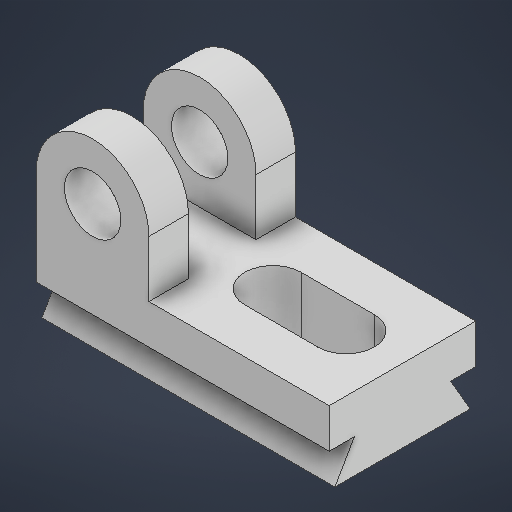
# Autodesk Inventor part: Pieza3
Saved by Autodesk Inventor 2026 (Build 300175000, 175)
## iProperties
Created: 2025-03-28
Part Number: Pieza3
Material: Genérico
Document SubType Name: Modeling
Designer: LabB305
Density: 1 g/cm^3
Appearance: Valor por defecto
Author: LabB305
Autodesk Inventor part; units mm, degrees
ref_plane "YZ Plane" through (0, 0, 0) normal (1, 0, 0) x (0, 1, 0)
ref_plane "XZ Plane" through (0, 0, 0) normal (0, 1, 0) x (-1, 0, 0)
ref_plane "XY Plane" through (0, 0, 0) normal (0, 0, 1) x (1, 0, 0)
sketch "Boceto1" plane through (0, 0, 0) normal (0, 1, 0) x (-1, 0, 0)
  point P0 (0, 0)
sketch "Boceto2" plane through (0, 0, 0) normal (1, 0, 0) x (0, 1, 0)
  line L0 (0, 0) -> (0, 12)
  line L1 (0, 0) -> (0, -12)
  line L2 (0, 0) -> (6, 0)
  line L3 (6, 0) -> (13, 0)
  line L4 (0, 12) -> (6, 8.5359)
  line L5 (0, 12) -> (6.9282, 12) construction
  line L6 (13, 0) -> (13, 13)
  line L7 (6, 8.5359) -> (6, 13)
  line L8 (6, 13) -> (13, 13)
  line L9 (13, 13) -> (33, 13)
  line L10 (33, 13) -> (33, 6)
  line L11 (33, 6) -> (13, 6)
  line L12 (0, 0) -> (0, -12)
  line L13 (0, -12) -> (6, -8.5359)
  line L14 (0, -12) -> (6.9282, -12) construction
  line L15 (13, 0) -> (13, -13)
  line L16 (6, -8.5359) -> (6, -13)
  line L17 (6, -13) -> (13, -13)
  line L18 (13, -13) -> (33, -13)
  line L19 (33, -13) -> (33, -6)
  line L20 (33, -6) -> (13, -6)
  dimension "d0" = 12
  dimension "d1" = 12
  dimension "d2" = 6
  dimension "d3" = 7
  dimension "d4" = 30
  dimension "d5" = 13
  dimension "d6" = 20
  dimension "d7" = 7
  constraints: 42 end point, 7 symmetric about line, 4 vertical, 3 horizontal, 3 perpendicular, 3 point on line, 1 equal length
  measures "d0" distance of L0.start L0.end
  measures "d1" distance of L0.start L1.end
  measures "d2" distance of L0.start L2.end
  measures "d3" distance of L2.end L3.end
  measures "d4" angle of L4 L5
  measures "d5" distance of L3.end L6.end
  measures "d6" distance of L6.end L9.end
  measures "d7" distance of L9.end L10.end
extrude "Extrusión1" add sketch "Boceto2" along normal blind 52 contours L2 L3 L15 L17 L16 L13 L1 | L0 L4 L7 L8 L6 L3 L2
sketch "Boceto3" plane through (0, 13, 13) normal (0, 1, 0) x (1, 0, 0)
  line L0 (52, 1) -> (52, 25) projected
  line L1 (52, 13) -> (42, 13)
  line L2 (42, 13) -> (29, 13)
  circle A0 centre (29, 13) radius 5
  circle A1 centre (42, 13) radius 5
  line L3 (29, 8) -> (42, 8)
  line L4 (29, 18) -> (42, 18)
  point P0 (0, 13)
  dimension "d10" = 10
  dimension "d11" = 13
  dimension "d12" = 10
  dimension "d13" = 10
  constraints: 8 end point, 4 point on circle, 2 centre point, 2 coincident, 2 tangent, 1 horizontal, 1 midpoint, 1 parallel, 1 point on line
  measures "d10" distance of L1.start L1.end
  measures "d11" distance of L1.end L2.end
  measures "d12" diameter of A0
  measures "d13" diameter of A1
extrude "Extrusión2" cut sketch "Boceto3" against normal blind 20
sketch "Boceto4" plane through (0, 13, 13) normal (0, 1, 0) x (1, 0, 0)
  line L0 (0, 0) -> (52, 0) projected
  line L1 (0, 0) -> (20, 0)
  line L2 (20, 0) -> (20, 7)
  line L3 (20, 7) -> (0, 7)
  line L4 (0, 1) -> (0, 25) projected
  line L5 (0, 13) -> (20, 13)
  line L6 (20, 26) -> (20, 19)
  line L7 (20, 19) -> (0, 19)
  line L8 (20, 26) -> (0, 26)
  line L9 (0, 26) -> (0, 19)
  line L10 (20, 0) -> (0, 0)
  line L11 (0, 0) -> (0, 7)
  dimension "d16" = 20
  dimension "d17" = 7
  constraints: 20 end point, 3 collinear, 3 symmetric about line, 2 horizontal, 2 perpendicular, 2 point on line
  measures "d16" distance of L0.start L1.end
  measures "d17" distance of L1.end L2.end
extrude "Extrusión3" add sketch "Boceto4" along normal blind 20
sketch "Boceto5" plane through (52, 6, -13) normal (0, 0, -1) x (-1, 0, 0)
  line L0 (32, 7) -> (42, 7)
  line L1 (52, 7) -> (32, 7) projected
  line L2 (42, 7) -> (42, 17)
  circle A0 centre (42, 17) radius 5
  point P0 (52, -6)
  dimension "d20" = 10
  dimension "d21" = 10
  dimension "d22" = 10
  constraints: 4 end point, 1 centre point, 1 coincident, 1 midpoint, 1 vertical
  measures "d20" distance of L0.start L0.end
  measures "d21" distance of L0.end L2.end
  measures "d22" diameter of A0
extrude "Extrusión4" cut sketch "Boceto5" against normal blind 30
fillet "Empalme1" radius 10 4 edges at (20, 33, 9.5) (20, 33, -9.5) (0, 33, 9.5) (0, 33, -9.5)
